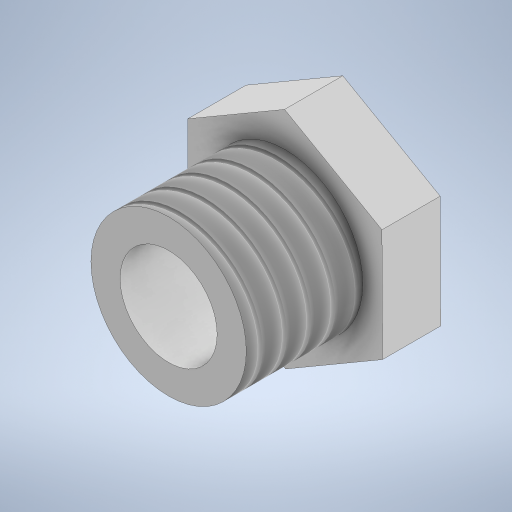
# Autodesk Inventor part: Hudson 1-57
Saved by Autodesk Inventor 2024.2 (Build 282272000, 272)
## iProperties
Created: 2024-10-06
Part Number: Hudson 1-57
Material: Genérico
Document SubType Name: Modeling
Designer: Monica Mora
Density: 1 g/cm^3
Appearance: Valor por defecto
Author: Monica Mora
Autodesk Inventor part; units mm, degrees
ref_plane "YZ Plane" through (0, 0, 0) normal (1, 0, 0) x (0, 1, 0)
ref_plane "XZ Plane" through (0, 0, 0) normal (0, 1, 0) x (-1, 0, 0)
ref_plane "XY Plane" through (0, 0, 0) normal (0, 0, 1) x (1, 0, 0)
sketch "Boceto1" plane through (0, 0, 0) normal (0, 0, 1) x (1, 0, 0)
  line L0 (5.0141, -2.8621) -> (0.0284, -5.7734)
  line L1 (0.0284, -5.7734) -> (-4.9858, -2.9113)
  line L2 (-4.9858, -2.9113) -> (-5.0141, 2.8621)
  line L3 (-5.0141, 2.8621) -> (-0.0284, 5.7734)
  line L4 (-0.0284, 5.7734) -> (4.9858, 2.9113)
  line L5 (4.9858, 2.9113) -> (5.0141, -2.8621)
  point P0 (0, 0)
  point P1 (0, 0)
  dimension "d0" = 10
  constraints: 12 end point, 1 coincident, 13 other
  measures "d0" distance between parallel lines of L5 L2
extrude "Extrusión1" add sketch "Boceto1" along normal blind 3
sketch "Boceto2" plane through (0, 0, 3) normal (0, 0, 1) x (1, 0, 0)
  circle A0 centre (0, 0) radius 4
  circle A1 centre (0, 0) radius 2.5
  dimension "d3" = 8
  dimension "d4" = 5
  constraints: 2 centre point, 2 coincident
  measures "d3" diameter of A0
  measures "d4" diameter of A1
extrude "Extrusión2" add sketch "Boceto2" along normal blind 6 contours A0 | A1
sketch "Boceto3" plane through (0, 0, 9) normal (0, 0, 1) x (1, 0, 0)
  point P0 (0, 0)
  point P1 (0, 0)
  constraints: 1 coincident
hole "Agujero1" at (0, 0, 9) direction (0, 0, -1) diameter 5 depth 7
thread "Rosca1" size "M8x1.25" class "6g" standard "ANSI Metric M Profile" length 18.5
